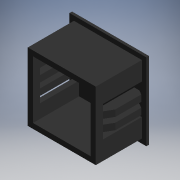
# Autodesk Inventor part: SLZ_63_Abdeck_Stoepsel#
Saved by Autodesk Inventor 2017.3 (Build 213256000, 256)
## iProperties
Part Number: SLZ_63_Abdeck_Stoepsel#
Material: Generic
Catalog Web Link: www.cadenas.de
Description: Stöpsel_SLZ63-Control-Tec
Vendor: ROSEKRIEGER
Document SubType Name: Modeling
Designer: partserver
Manufacturer: ROSEKRIEGER
Mass: 0.799069 g
Surface Area: 14.419 cm^2
Volume: 0.799069 cm^3
Density: 1 g/cm^3
Appearance: PSOLRGB-64-64-64
Category: PARTsolutions
Company: ROSEKRIEGER
Title: SLZ_63_Abdeck_Stoepsel#
Author: Cadenas PARTsolutions
Comments: Control-Tec
PSOL_IDENT_0: {$CADENAS_DATA\23d-libs\rose_krieger\linearkomponenten\pool_lineartechnik\_hubsaeule_zyliinder\elekt
PSOL_IDENT_1: rozylinder\elekzyl_slz63\parts\slz63_plfl_abdeck_stoepsel.prj},193 {VTYP=3D},{NB=SLZ_63_Abdeck_Stoep
PSOL_IDENT_2: sel#},{LINA=SLZ_63_Abdeck_Stoepsel#},{NN=Stöpsel_SLZ63},{DATE=02.12.2020 11:16:21},{GEOMDATE=22.06.2
PSOL_IDENT_3: 016 13:22:52},{VERSION=},{LINEID=10},{WBVAR=},{WBNUMERIC=}  {NB=SLZ_63_Abdeck_Stoepsel#},{LINA=SLZ_6
PSOL_IDENT_4: 3_Abdeck_Stoepsel#},{KT=DUMMY},{IDNR=},{CODE=TQ3},{ARTIKEL=Elektrozylinder },{TYPE=SLZ 63 KG P PL},{
PSOL_IDENT_5: BEST=SLZ_63_Abdeck_Stoepsel},{VARIANTE=PL},{SPINDEL=KG 25x10},{SPINDELCODE=3.000},{SCHUTZARTVIS=IP54
PSOL_IDENT_6: },{SCHUTZART=1},{HUB1=0,[0:100]},{HINWEINBAUX=Hub + 288,5 mm},{DUMMYDURCH=10.000},{DUMMYLAENG=20.000
PSOL_IDENT_7: },{HILFEHUB=105},{LAENDOPPROFIL=184.500},{RF=1.000},{GRUNDKOE=288.500},{A=100},{B=80},{C=100},{D=125
PSOL_IDENT_8: },{E=238},{F=40},{G=M16x1.5},{H=104},{K=125},{L=105},{M=48},{N=56.5},{O=86},{P=18.5},{PPATH=sbl_lz70
PSOL_IDENT_9: p_plfl.prj}
NB: SLZ_63_Abdeck_Stoepsel#
NN: Stöpsel_SLZ63
NT: Control-Tec
NBSYN: $BEST.#
LINA: SLZ_63_Abdeck_Stoepsel#
CATALOG: RK Rose+Krieger
CODE: TQ3
ARTIKEL: Elektrozylinder
TYPE: SLZ 63 KG P PL
BEST: SLZ_63_Abdeck_Stoepsel
VARIANTE: PL
SPINDEL: KG 25x10
SPINDELCODE: 3
SCHUTZARTVIS: IP54
SCHUTZART: 1
HUB1: 0,[0:100]
HINWEINBAUX: Hub + 288,5 mm
DUMMYDURCH: 10
DUMMYLAENG: 20
HILFEHUB: 105
LAENDOPPROFIL: 184.5
RF: 1
GRUNDKOE: 288.5
A: 100
B: 80
C: 100
D: 125
E: 238
F: 40
G: M16x1.5
H: 104
K: 125
L: 105
M: 48
N: 56.5
O: 86
P: 18.5
PPATH: sbl_lz70p_plfl.prj
SUPPLIER: ROSEKRIEGER
ARTICLENO: SLZ_63_Abdeck_Stoepsel#
BOMINFO: SLZ_63_Abdeck_Stoepsel#
CREATOR: CADENAS GmbH
Autodesk Inventor part; units mm, degrees
sketch "Sketch_1" plane through (0, 0, 0) normal (0, 0, 1) x (1, 0, 0)
  line L0 (-7.5, -1.5) -> (-7.5, -2)
  line L1 (-7.5, -2) -> (7.5, -2)
  line L2 (7.5, -2) -> (7.5, -1.5)
  line L3 (7.5, -1.5) -> (6, 0)
  line L4 (6, 0) -> (-6, 0)
  line L5 (-6, 0) -> (-7.5, -1.5)
  constraints: 12 end point
extrude "Extrusion1" add sketch "Sketch_1" along normal mid plane 15
sketch "Sketch_2" plane through (0, 0, 0) normal (1, 0, 0) x (0, 0, -1)
  line L0 (-7.5, -1.5) -> (-6, 0)
  line L1 (-6, 0) -> (6, 0)
  line L2 (6, 0) -> (7.5, -1.5)
  line L3 (7.5, -1.5) -> (7.5, 3.5)
  line L4 (7.5, 3.5) -> (-7.5, 3.5)
  line L5 (-7.5, 3.5) -> (-7.5, -1.5)
  constraints: 12 end point
extrude "Extrusion2" cut sketch "Sketch_2" along normal mid plane 15
sketch "Sketch_3" plane through (0, -2, 0) normal (0, 1, 0) x (1, 0, 0)
  line L0 (-6.625, -6.625) -> (6.625, -6.625)
  line L1 (6.625, -6.625) -> (6.625, 6.625)
  line L2 (6.625, 6.625) -> (-6.625, 6.625)
  line L3 (-6.625, 6.625) -> (-6.625, -6.625)
  line L4 (-5.625, -5.625) -> (5.625, -5.625)
  line L5 (5.625, -5.625) -> (5.625, 5.625)
  line L6 (5.625, 5.625) -> (-5.625, 5.625)
  line L7 (-5.625, 5.625) -> (-5.625, -5.625)
  constraints: 16 end point
extrude "Extrusion3" add sketch "Sketch_3" against normal blind 9
sketch "Sketch_4" plane through (0, 0, 0) normal (0, 0, 1) x (1, 0, 0)
  line L0 (-7.5, -9.6) -> (7.5, -9.6)
  line L1 (7.5, -9.6) -> (7.5, -2)
  line L2 (7.5, -2) -> (-7.5, -2)
  line L3 (-7.5, -2) -> (-7.5, -9.6)
  constraints: 8 end point
extrude "Extrusion4" cut sketch "Sketch_4" along normal mid plane 6
sketch "Sketch_6" plane through (0, 0, 1.125) normal (0, 0, 1) x (1, 0, 0)
  line L0 (5.625, -2.5) -> (5.625, -9.6)
  line L1 (5.625, -9.6) -> (6.625, -9.6)
  line L2 (6.625, -9.6) -> (7.505, -8.0758)
  line L3 (7.505, -8.0758) -> (7.505, -3.0081)
  line L4 (7.505, -3.0081) -> (6.625, -2.5)
  line L5 (6.625, -2.5) -> (5.625, -2.5)
  constraints: 12 end point
extrude "Extrusion5" add sketch "Sketch_6" along normal mid plane 1.25
sketch "Sketch_7" plane through (0, 0, 1.125) normal (0, 0, 1) x (1, 0, 0)
  line L0 (-7.505, -3.0081) -> (-7.505, -8.0758)
  line L1 (-7.505, -8.0758) -> (-6.625, -9.6)
  line L2 (-6.625, -9.6) -> (-5.625, -9.6)
  line L3 (-5.625, -9.6) -> (-5.625, -2.5)
  line L4 (-5.625, -2.5) -> (-6.625, -2.5)
  line L5 (-6.625, -2.5) -> (-7.505, -3.0081)
  constraints: 12 end point
extrude "Extrusion6" add sketch "Sketch_7" along normal mid plane 1.25
sketch "Sketch_8" plane through (0, 0, -1.125) normal (0, 0, 1) x (1, 0, 0)
  line L0 (5.625, -2.5) -> (5.625, -9.6)
  line L1 (5.625, -9.6) -> (6.625, -9.6)
  line L2 (6.625, -9.6) -> (7.505, -8.0758)
  line L3 (7.505, -8.0758) -> (7.505, -3.0081)
  line L4 (7.505, -3.0081) -> (6.625, -2.5)
  line L5 (6.625, -2.5) -> (5.625, -2.5)
  constraints: 12 end point
extrude "Extrusion7" add sketch "Sketch_8" along normal mid plane 1.25
sketch "Sketch_9" plane through (0, 0, -1.125) normal (0, 0, 1) x (1, 0, 0)
  line L0 (-7.505, -3.0081) -> (-7.505, -8.0758)
  line L1 (-7.505, -8.0758) -> (-6.625, -9.6)
  line L2 (-6.625, -9.6) -> (-5.625, -9.6)
  line L3 (-5.625, -9.6) -> (-5.625, -2.5)
  line L4 (-5.625, -2.5) -> (-6.625, -2.5)
  line L5 (-6.625, -2.5) -> (-7.505, -3.0081)
  constraints: 12 end point
extrude "Extrusion8" add sketch "Sketch_9" along normal mid plane 1.25
ref_plane "ABDECKSTOEPSEL_XY" through (0, 0, -7.5) normal (0, 0, -1) x (1, 0, 0)
ref_plane "ABDECKSTOEPSEL_YZ" through (0, 0, -7.5) normal (1, 0, 0) x (0, -1, 0)
ref_plane "ABDECKSTOEPSEL_ZX" through (0, 0, -7.5) normal (0, -1, 0) x (0, 0, -1)
body "Solid1"
